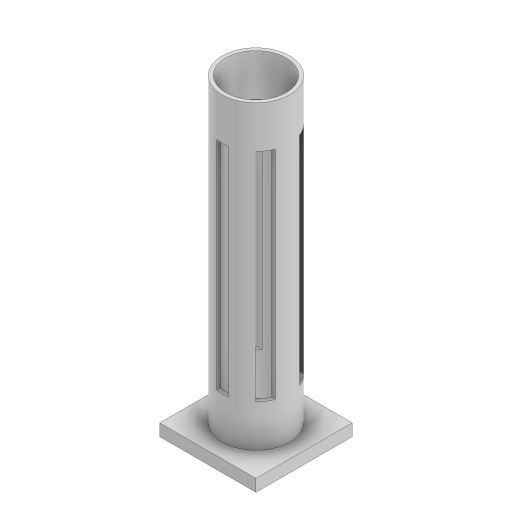
# Autodesk Inventor part: TUBO CONTENEDOR
Saved by Autodesk Inventor 2024 (Build 280153000, 153)
## iProperties
Created: 2024-06-30
Part Number: TUBO CONTENEDOR
Material: Generic
Document SubType Name: Modeling
Designer: Jhuliams
Density: 1 g/cm^3
Appearance: Default
Author: Jhuliams
Autodesk Inventor part; units mm, degrees
ref_plane "YZ Plane" through (0, 0, 0) normal (1, 0, 0) x (0, 1, 0)
ref_plane "XZ Plane" through (0, 0, 0) normal (0, 1, 0) x (-1, 0, 0)
ref_plane "XY Plane" through (0, 0, 0) normal (0, 0, 1) x (1, 0, 0)
sketch "Sketch1" plane through (0, 0, 0) normal (0, 1, 0) x (-1, 0, 0)
  circle A0 centre (0, 0) radius 25
  circle A1 centre (0, 0) radius 28
  dimension "d0" = 50
  dimension "d1" = 56
  constraints: 2 centre point, 2 coincident
  measures "d0" diameter of A0
  measures "d1" diameter of A1
extrude "Extrusion1" add sketch "Sketch1" along normal blind 250
sketch "Sketch2" plane through (0, 0, 0) normal (1, 0, 0) x (0, 1, 0)
  line L0 (0, 0) -> (0, 15)
  line L1 (0, -28) -> (0, 28) projected
  line L2 (0, 15) -> (125, 15)
  line L3 (215, 20) -> (35, 20)
  line L4 (35, 20) -> (35, 10)
  line L5 (35, 10) -> (215, 10)
  line L6 (215, 10) -> (215, 20)
  line L7 (215, 20) -> (35, 10) construction
  line L8 (35, 20) -> (215, 10) construction
  line L9 (0, 0) -> (25, 0)
  line L10 (215, -20) -> (35, -20)
  line L11 (35, -20) -> (35, -10)
  line L12 (35, -10) -> (215, -10)
  line L13 (215, -10) -> (215, -20)
  line L14 (215, -20) -> (35, -10) construction
  line L15 (35, -20) -> (215, -10) construction
  point P0 (125, -15)
  dimension "d4" = 15
  dimension "d5" = 125
  dimension "d6" = 180
  dimension "d7" = 10
  dimension "d8" = 25
  constraints: 30 end point, 5 symmetric about line, 3 horizontal, 2 midpoint, 2 parallel, 1 perpendicular, 1 point on line
  measures "d4" distance of L0.start L0.end
  measures "d5" distance of L0.end L2.end
  measures "d6" distance of L5.end L4.end
  measures "d7" distance of L4.end L3.end
  measures "d8" distance of L0.start L9.end
extrude "Extrusion2" cut sketch "Sketch2" along normal mid plane 100
sketch "Sketch4" plane through (0, 0, 0) normal (0, 0, 1) x (1, 0, 0)
  line L0 (0, 0) -> (0, 125)
  line L1 (-5, 215) -> (5, 215)
  line L2 (5, 215) -> (5, 35)
  line L3 (5, 35) -> (-5, 35)
  line L4 (-5, 35) -> (-5, 215)
  line L5 (-5, 215) -> (5, 35) construction
  line L6 (5, 215) -> (-5, 35) construction
  dimension "d11" = 125
  dimension "d12" = 10
  dimension "d13" = 180
  constraints: 14 end point, 2 midpoint, 2 parallel, 1 horizontal, 1 perpendicular, 1 vertical
  measures "d11" distance of L0.start L0.end
  measures "d12" distance of L2.end L3.end
  measures "d13" distance of L1.end L2.end
extrude "Extrusion3" cut sketch "Sketch4" along normal mid plane 100
sketch "Sketch5" plane through (0, 0, 0) normal (0, -1, 0) x (1, 0, 0)
  line L0 (-40, 40) -> (40, 40)
  line L1 (40, 40) -> (40, -40)
  line L2 (40, -40) -> (-40, -40)
  line L3 (-40, -40) -> (-40, 40)
  line L4 (-40, 40) -> (40, -40) construction
  line L5 (40, 40) -> (-40, -40) construction
  circle A0 centre (0, 0) radius 28
  dimension "d16" = 80
  dimension "d17" = 80
  dimension "d18" = 56
  constraints: 12 end point, 2 midpoint, 2 parallel, 1 centre point, 1 coincident, 1 horizontal, 1 perpendicular
  measures "d16" distance of L1.end L2.end
  measures "d17" distance of L0.end L1.end
  measures "d18" diameter of A0
extrude "Extrusion4" add sketch "Sketch5" along normal blind 10
body "Solid1"
